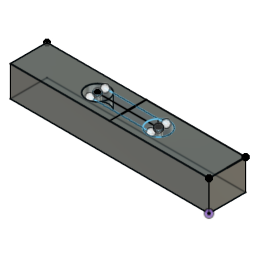
hexbug_2.5cm_mold_final (Autodesk Fusion 360 design; units mm, degrees)
Autodesk Fusion 360 part; units mm, degrees
sketch "Sketch1" plane through (0, 0, 0) normal (0, 0, 1) x (1, 0, 0)
  line L0 (0, 0) -> (-65, 0)
  line L1 (-65, 0) -> (-65, 12)
  line L2 (-65, 12) -> (0, 12)
  line L3 (0, 12) -> (0, 0)
  dimension "d1" = 12
  dimension "d2" = 65
  constraint horizontal L0
  constraint vertical L1
  constraint horizontal L2
  constraint vertical L3
  constraint coincident L0.start L3.end
  measures "d1" distance of L0.start L2.end
  measures "d2" distance of L0.start L0.end
extrude "Extrude1" add sketch "Sketch1" along normal blind 10
sketch "Sketch2" plane through (0, 0, 10) normal (0, 0, 1) x (-1, 0, 0)
  line L0 (0, -12) -> (65, -12)
  line L1 (65, -12) -> (65, 0)
  line L2 (65, 0) -> (0, 0)
  line L3 (0, 0) -> (0, -12)
  line L4 (0, -12) -> (0, -6)
  line L5 (0, -12) -> (32.5, -12)
  line L6 (32.5, -12) -> (32.5, 0)
  line L7 (32.5, -12) -> (32.5, -6)
  line L8 (32.5, -6) -> (22.5, -6)
  line L9 (32.5, -6) -> (42.5, -6)
  line L10 (32.5, -6) -> (32.5, -3.5)
  line L11 (32.5, -6) -> (32.5, -8.5)
  line L12 (32.5, -8.5) -> (22.5, -8.5)
  line L13 (32.5, -3.5) -> (22.5, -3.5)
  line L14 (32.5, -3.5) -> (42.5, -3.5)
  line L15 (42.5, -8.5) -> (32.5, -8.5)
  circle A0 centre (42.5, -6) radius 1
  circle A1 centre (22.5, -6) radius 1
  circle A2 centre (42.5, -6) radius 3.65
  circle A3 centre (22.5, -6) radius 3.65
  line L16 (0, 0) -> (65, 0)
  line L17 (65, 0) -> (65, -12)
  line L18 (65, -12) -> (0, -12)
  line L19 (0, -12) -> (0, 0)
  dimension "d5" = 10
  dimension "d7" = 10
  dimension "d9" = 2.5
  dimension "d10" = 2.5
  dimension "d11" = 2
  dimension "d12" = 2
  dimension "d15" = 7.3
  dimension "d16" = 7.3
  constraint coincident L0.start L3.end
  constraint midpoint L3 L4.end
  constraint midpoint L0 L5.end
  constraint midpoint L2 L6.end
  constraint midpoint L6 L7.end
  constraint perpendicular L6 L8
  constraint perpendicular L6 L9
  constraint perpendicular L8 L10
  constraint perpendicular L8 L11
  constraint coincident L9.end A0.centre
  constraint horizontal L16
  constraint vertical L17
  constraint horizontal L18
  constraint vertical L19
  constraint coincident L0.end L1.start
  constraint coincident L2.end L3.start
  measures "d5" distance of L7.end L8.end
  measures "d7" distance of L7.end L9.end
  measures "d9" distance of L7.end L10.end
  measures "d10" distance of L7.end L11.end
  measures "d11" diameter of A0
  measures "d12" diameter of A1
  measures "d15" diameter of A2
  measures "d16" diameter of A3
extrude "Extrude3" cut sketch "Sketch2" against normal blind 5 contours L6 L7 L8 L11 L12 A3 | L6 L7 L9 L11 L15 A2 | L6 L8 L10 L13 A3 | L6 L9 L10 L14 A2 | A3 | A2
extrude "Extrude5" [suppressed]
sketch "Sketch4" plane through (0, 12, 0) normal (0, 1, 0) x (-1, 0, 0)
  line L0 (0, 0) -> (65, 0)
  line L1 (65, 0) -> (65, 20)
  line L2 (65, 20) -> (0, 20)
  line L3 (0, 20) -> (0, 0)
  line L4 (0, 20) -> (0, 10)
  line L5 (0, 10) -> (65, 10)
  constraint coincident L2.end L3.start
  constraint midpoint L3 L4.end
  constraint midpoint L1 L5.end
split "Split1" [suppressed]
sketch "Sketch5" plane through (0, 0, 10) normal (0, 0, 1) x (-1, 0, 0)
  line L0 (25.1594, -3.5) -> (39.8406, -3.5)
  arc A0 (39.8406, -8.5) -> (39.8406, -3.5) centre (42.5, -6) ccw
  line L1 (39.8406, -8.5) -> (25.1594, -8.5)
  arc A1 (25.1594, -3.5) -> (25.1594, -8.5) centre (22.5, -6) ccw
  line L2 (65, 0) -> (0, 0)
  line L3 (0, 0) -> (0, -12)
  line L4 (0, -12) -> (65, -12)
  line L5 (65, -12) -> (65, 0)
  line L6 (0, 0) -> (0, -12)
  line L7 (0, -6) -> (5, -6)
  circle A2 centre (5, -6) radius 1.25
  line L8 (65, -6) -> (60, -6)
  circle A3 centre (60, -6) radius 1.25
  dimension "d28" = 5
  dimension "d29" = 2.5
  dimension "d30" = 5
  dimension "d31" = 2.5
  constraint coincident L2.end L3.start
  constraint coincident L3.end L4.start
  constraint midpoint L3 L7.start
  constraint perpendicular L3 L7
  constraint coincident L7.end A2.centre
  constraint midpoint L5 L8.start
  constraint perpendicular L5 L8
  constraint coincident L8.end A3.centre
  measures "d28" distance of L7.start L7.end
  measures "d29" diameter of A2
  measures "d30" distance of L8.start L8.end
  measures "d31" diameter of A3
extrude "Extrude6" [suppressed]
sketch "Sketch6" plane through (0, 0, 10) normal (0, 0, -1) x (1, 0, 0)
  line L0 (0, 0) -> (-65, 0)
  line L1 (-65, 0) -> (-65, -12)
  line L2 (-65, -12) -> (0, -12)
  line L3 (0, -12) -> (0, 0)
  line L4 (0, -6) -> (-5, -6)
  circle A0 centre (-5, -6) radius 1.25
  line L5 (-65, 0) -> (-65, -6)
  line L6 (-65, -6) -> (-60, -6)
  circle A1 centre (-60, -6) radius 1.25
  dimension "d34" = 5
  dimension "d35" = 2.5
  dimension "d36" = 5
  dimension "d37" = 2.5
  constraint midpoint L3 L4.start
  constraint perpendicular L3 L4
  constraint coincident L4.end A0.centre
  constraint coincident L0.end L1.start
  constraint midpoint L1 L5.end
  constraint perpendicular L1 L6
  constraint coincident L6.end A1.centre
  measures "d34" distance of L4.start L4.end
  measures "d35" diameter of A0
  measures "d36" distance of L5.end L6.end
  measures "d37" diameter of A1
extrude "Extrude7" [suppressed]
hole "Hole2" [suppressed]
extrude "Extrude2" [suppressed]
